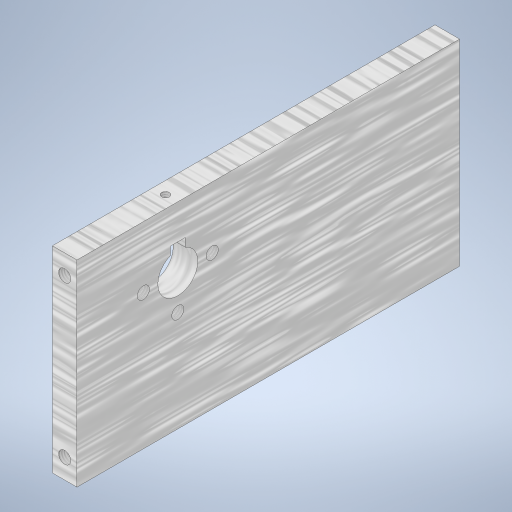
# Autodesk Inventor part: shoulder1_verticval_cover
Saved by Autodesk Inventor 2024 (Build 280153000, 153)
## iProperties
Created: 2025-08-06
Part Number: shoulder1_verticval_cover
Material: アルミニウム 5052
Document SubType Name: Modeling
Designer: HosodaLab2
Density: 2.68 g/cm^3
Appearance: サテン - ブラシ仕上げ 重厚
個数: 2
Author: HosodaLab2
Autodesk Inventor part; units mm, degrees
note: some values were not read from the file. Chosen so that the rebuilt part matches the saved one: direction of "穴8".
ref_plane "YZ Plane" through (0, 0, 0) normal (1, 0, 0) x (0, 1, 0)
ref_plane "XZ Plane" through (0, 0, 0) normal (0, 1, 0) x (-1, 0, 0)
ref_plane "XY Plane" through (0, 0, 0) normal (0, 0, 1) x (1, 0, 0)
sketch "スケッチ2" plane through (0, 0, 0) normal (0, 1, 0) x (-1, 0, 0)
  line L0 (0, 0) -> (-77.8, 0)
  line L1 (-77.8, 0) -> (-77.8, -40)
  line L2 (-77.8, -40) -> (0, -40)
  line L3 (0, -40) -> (0, 0)
  dimension "d0" = 77.8
  dimension "d1" = 40
  constraints: 8 end point, 2 parallel, 1 horizontal, 1 perpendicular
  measures "d0" distance of L2.end L1.end
  measures "d1" distance of L1.end L0.end
extrude "押し出し1" add sketch "スケッチ2" along normal blind 5
sketch "スケッチ4" plane through (0, 0, -40) normal (-1, 0, 0) x (0, 0, 1)
  line L0 (0, 0) -> (0, 5) construction
  line L1 (0, 2.5) -> (40, 2.5) construction
  line L2 (40, 0) -> (40, 5) construction
  point P0 (4, 2.5)
  point P1 (36, 2.5)
  dimension "d4" = 4
  dimension "d5" = 4
  constraints: 2 end point, 2 midpoint, 2 point on line
  measures "d4" distance from line of L2 point (36, 2.5)
  measures "d5" distance from line of point (4, 2.5) L0
hole "穴1" at (0, 2.5, -36) at (0, 2.5, -4) direction (1, 0, 0) diameter 2.459 depth 12 thread size "M3x0.5" class "6H" standard "ISO Metric profile"
sketch "スケッチ5" plane through (77.8, 0, 0) normal (1, 0, 0) x (0, 0, -1)
  line L0 (0, 0) -> (0, 5) construction
  line L1 (0, 2.5) -> (39.9198, 2.5) construction
  circle A0 centre (4, 2.5) radius 1.2295 construction
  circle A1 centre (36, 2.5) radius 1.2295 projected
  point P0 (4, 2.5)
  point P1 (36, 2.5)
  constraints: 2 coincident, 2 end point, 1 horizontal, 1 midpoint
hole "穴2" at (77.8, 2.5, -4) at (77.8, 2.5, -36) direction (-1, 0, 0) diameter 2.459 depth 13 thread size "M3x0.5" class "6H" standard "ISO Metric profile"
sketch "スケッチ6" plane through (0, 5, 0) normal (0, 1, 0) x (1, 0, 0)
  line L0 (77.8, 0) -> (77.8, 40) construction
  line L1 (0, 40) -> (0, 0) construction
  line L2 (0, 0) -> (77.8, 0) construction
  point P0 (57.3, 12.5)
  dimension "d20" = 20.5
  dimension "d21" = 12.5
  measures "d20" distance from line of L0 point (57.3, 12.5)
  measures "d21" distance from line of L2 point (57.3, 12.5)
hole "穴3" at (57.3, 5, -12.5) direction (0, -1, 0) diameter 8.1 end through all
sketch "スケッチ7" plane through (0, 5, 0) normal (0, 1, 0) x (1, 0, 0)
  line L0 (77.8, 0) -> (77.8, 40) construction
  line L1 (77.8, 28.3) -> (0, 28.3) construction
  line L2 (0, 40) -> (0, 0) construction
  circle A0 centre (57.3, 12.5) radius 4.05 construction
  point P0 (67.8, 28.3)
  point P1 (46.8, 28.3)
  dimension "d29" = 15.8
  dimension "d30" = 10.5
  dimension "d31" = 10.5
  constraints: 4 point on line, 2 end point, 1 horizontal
  measures "d29" distance from line of L1 A0.centre
  measures "d30" horizontal distance of point (67.8, 28.3) A0.centre
  measures "d31" horizontal distance of point (46.8, 28.3) A0.centre
hole "穴4" [suppressed]
sketch "スケッチ11" plane through (0, 5, 0) normal (0, 1, 0) x (1, 0, 0)
  circle A0 centre (57.3, 12.5) radius 4.05 projected
  line L0 (55.8, 7.05) -> (58.8, 7.05)
  line L1 (58.8, 7.05) -> (58.8, 8.45)
  line L2 (58.8, 8.45) -> (55.8, 8.45)
  line L3 (55.8, 8.45) -> (55.8, 7.05)
  line L4 (55.8, 8.45) -> (55.8, 8.738)
  line L5 (58.8, 8.45) -> (58.8, 8.738)
  point P0 (0, 0)
  point P1 (57.3, 8.45)
  dimension "d68" = 1.4
  dimension "d69" = 3
  constraints: 12 end point, 3 parallel, 2 point on circle, 1 horizontal, 1 midpoint, 1 perpendicular, 1 tangent, 1 vertical, 1 vertical alignment
  measures "d68" distance of L0.end L1.end
  measures "d69" distance of L1.end L2.end
extrude "押し出し3" cut sketch "スケッチ11" against normal through all contours A0 L2 L4 | L5 L2 A0 | L2 L1 L0 L3
sketch "スケッチ8" plane through (0, 5, 0) normal (0, 1, 0) x (1, 0, 0)
  arc A0 (58.8, 8.738) -> (55.8, 8.738) centre (57.3, 12.5) ccw construction
  circle A1 centre (57.3, 12.5) radius 7 construction
  point P0 (0, 0)
  point P1 (57.3, 19.5)
  point P2 (50.3, 12.5)
  point P3 (64.3, 12.5)
  dimension "d39" = 14
  constraints: 3 point on circle, 2 horizontal alignment, 1 centre point, 1 coincident, 1 vertical alignment
  measures "d39" diameter of A1
hole "穴5" at (57.3, 5, -19.5) at (50.3, 5, -12.5) at (64.3, 5, -12.5) direction (0, -1, 0) diameter 2.459 end through all thread size "M3x0.5" class "6H" standard "ISO Metric profile"
sketch "スケッチ9" plane through (0, 5, 0) normal (0, 1, 0) x (1, 0, 0)
  circle A0 centre (57.3, 12.5) radius 4.05 projected
  line L0 (57.3, 12.5) -> (45.9478, 12.5) construction
  line L1 (51.85, 14) -> (53.25, 14)
  line L2 (53.25, 14) -> (53.25, 11)
  line L3 (53.25, 11) -> (51.85, 11)
  line L4 (51.85, 11) -> (51.85, 14)
  line L5 (51.85, 14) -> (53.25, 11) construction
  line L6 (53.25, 14) -> (51.85, 11) construction
  line L7 (53.25, 11) -> (53.538, 11)
  line L8 (53.25, 14) -> (53.538, 14)
  point P0 (0, 0)
  point P1 (52.55, 12.5)
  point P2 (53.25, 12.5)
  dimension "d56" = 1.4
  dimension "d57" = 0
  dimension "d58" = 3
  constraints: 18 end point, 4 horizontal, 3 midpoint, 2 parallel, 2 point on circle, 1 perpendicular, 1 point on line
  measures "d56" distance of L2.end L3.end
  measures "d57" distance edge to line of A0 L2
  measures "d58" distance between parallel lines of L1 L3
extrude "押し出し2" [suppressed]
sketch "スケッチ12" plane through (0, 5, 0) normal (0, 1, 0) x (1, 0, 0)
  arc A0 (58.8, 8.738) -> (55.8, 8.738) centre (57.3, 12.5) ccw projected
  point P0 (0, 0)
  point P1 (50.3, 12.5)
  point P2 (57.3, 5.5)
  point P3 (64.3, 12.5)
  point P4 (57.3, 19.5)
  dimension "d74" = 360
  dimension "d76" = 14
  constraints: 1 horizontal alignment, 5 other
  measures "d76" distance of point (57.3, 19.5) point (57.3, 5.5)
hole "穴7" [suppressed]
sketch "スケッチ13" plane through (0, 0, 0) normal (0, 0, 1) x (1, 0, 0)
  line L0 (58.8, 5) -> (55.8, 5) projected
  line L1 (77.8, 0) -> (77.8, 5) projected
  point P0 (0, 0)
  point P1 (57.3, 2.5)
  point P2 (57.3, 5)
  point P3 (77.8, 2.5)
  constraints: 2 midpoint, 1 horizontal alignment, 1 vertical alignment
hole "穴8" at (57.3, 2.5, 0) direction (0, 0, -1) diameter 1.567 depth 7.05 thread size "M2x0.4" class "6H" standard "ISO Metric profile"
